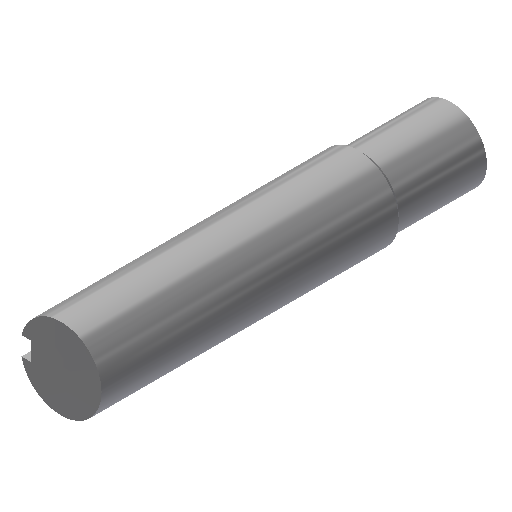
# Autodesk Inventor part: shaft
Saved by Autodesk Inventor 2022 (Build 260148000, 148)
## iProperties
Created: 2007-05-11
Part Number: shaft
Material: Steel, Mild
Document SubType Name: Modeling
Designer: LionelF
Density: 7.86 g/cm^3
Mass: 11720.6 g
Surface Area: 1167.38 cm^2
Volume: 1491.17 cm^3
Appearance: Steel
Author: LionelF
Autodesk Inventor part; units mm, degrees
ref_plane "YZ Plane" through (0, 0, 0) normal (1, 0, 0) x (0, 1, 0)
ref_plane "XZ Plane" through (0, 0, 0) normal (0, 1, 0) x (-1, 0, 0)
sketch "Sketch1" plane through (0, 0, 0) normal (0, 0, 1) x (1, 0, 0)
  circle A0 centre (0, 0) radius 27.7812
  dimension "d0" = 55.5625
  constraints: 1 centre point
  measures "d0" diameter of A0
extrude "Extrusion1" add sketch "Sketch1" along normal blind 266.7
ref_plane "Work Plane1" through (0, 0, 0) normal (0, 1, 0) x (0, 0, 1)
sketch "Sketch2" plane through (0, 0, 0) normal (0, 1, 0) x (0, 0, 1)
  line L0 (-53.34, 0) -> (320.04, 0) projected
  line L1 (0, -24.6062) -> (60.325, -24.6062)
  line L2 (60.325, -24.6062) -> (63.5, -27.7812)
  line L3 (0, -27.7812) -> (266.7, -27.7812) projected
  line L4 (0, -24.6062) -> (0, -27.7812)
  line L5 (0, 27.7812) -> (0, -27.7812) projected
  dimension "d4" = 24.6062
  dimension "d5" = 135
  dimension "d6" = 60.325
  constraints: 6 end point, 3 point on line, 1 parallel, 1 perpendicular
  measures "d4" distance between parallel lines of L1 L0
  measures "d5" angle of L1 L2
  measures "d6" distance of L1.start L1.end
revolve "Revolution1" cut sketch "Sketch2" angle 360 about axis through (0, 0, 0) along (0, 0, 1)
sketch "Sketch3" plane through (0, 0, 0) normal (0, 1, 0) x (0, 0, 1)
  line L0 (60.325, -24.6062) -> (0, -24.6062) projected
  line L1 (0, 24.6062) -> (0, -24.6062) projected
  line L2 (-127.1587, 0) -> (762.9525, 0) projected
  line L3 (0, -17.1768) -> (54.6612, -17.1767)
  arc A0 (85.725, -27.7812) -> (54.6612, -17.1767) centre (54.6612, -67.9767) ccw
  line L4 (60.325, 24.6062) -> (0, 24.6062) projected
  line L5 (63.5, -27.7812) -> (266.7, -27.7812) projected
  line L6 (63.5, -27.7812) -> (60.325, -24.6062)
  dimension "d8" = 50.8
  dimension "d9" = 41.783
  dimension "d10" = 85.725
  constraints: 4 end point, 2 point on circle, 2 point on line, 1 centre point, 1 parallel, 1 tangent
  measures "d8" radius of A0
  measures "d9" distance between parallel lines of L4 L3
  measures "d10" distance from line of L1 A0.start
extrude "Extrusion2" cut sketch "Sketch3" against normal mid plane 12.7
sketch "Sketch4" plane through (0, 0, 0) normal (0, 1, 0) x (0, 0, 1)
  line L0 (266.7, 27.7812) -> (266.7, -27.7812) projected
  line L1 (85.725, -27.7812) -> (266.7, -27.7812) projected
  line L2 (63.5, 27.7812) -> (266.7, 27.7812) projected
  line L3 (266.7, -20.4788) -> (165.1, -20.4788)
  arc A0 (165.1, -20.4788) -> (139.7, -27.7812) centre (165.1, -68.3039) ccw
  dimension "d13" = 101.6
  dimension "d14" = 127
  dimension "d15" = 48.26
  constraints: 2 end point, 2 point on circle, 2 point on line, 1 centre point, 1 parallel, 1 tangent
  measures "d13" distance of L3.start L3.end
  measures "d14" distance from line of A0.end L0
  measures "d15" distance between parallel lines of L2 L3
extrude "Extrusion3" cut sketch "Sketch4" against normal mid plane 12.7
body "Solid1"
